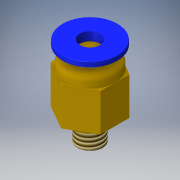
# Autodesk Inventor part: Bowden
Saved by Autodesk Inventor 2016 SP1 (Build 200210100, 210)
## iProperties
Created: 2015-12-27
Part Number: Bowden
Material: Generic
Document SubType Name: Modeling
Designer: Dirk Alferink
Density: 1 g/cm^3
Appearance: Gold
Author: Dirk Alferink
Autodesk Inventor part; units mm, degrees
ref_plane "YZ Plane" through (0, 0, 0) normal (1, 0, 0) x (0, 1, 0)
ref_plane "XZ Plane" through (0, 0, 0) normal (0, 1, 0) x (-1, 0, 0)
ref_plane "XY Plane" through (0, 0, 0) normal (0, 0, 1) x (1, 0, 0)
sketch "Sketch1" plane through (0, 0, 0) normal (0, 1, 0) x (-1, 0, 0)
  line L0 (0, 0) -> (2.5, 0)
  line L1 (2.5, 0) -> (2.5, 4)
  line L2 (2.5, 4) -> (4, 4)
  line L3 (4, 4) -> (4, 5)
  line L4 (4, 5) -> (0, 5)
  line L5 (0, 5) -> (0, 0)
  dimension "d0" = 2.5
  dimension "d1" = 4
  dimension "d2" = 1.5
  constraints: 12 end point, 4 perpendicular, 2 horizontal
  measures "d0" distance of L0.start L0.end
  measures "d1" distance of L0.end L1.end
  measures "d2" distance of L1.end L2.end
revolve "Revolution1" add sketch "Sketch1" angle 360 about axis through (0, 0, 5) along (0, 0, -1)
thread "Thread1" size "M5x0.8" class "6g" standard "ANSI Metric M Profile" full length
sketch "Sketch2" plane through (0, 0, 5) normal (0, 0, 1) x (1, 0, 0)
  line L0 (5, 2.8868) -> (5, -2.8868)
  line L1 (5, -2.8868) -> (0, -5.7735)
  line L2 (0, -5.7735) -> (-5, -2.8868)
  line L3 (-5, -2.8868) -> (-5, 2.8868)
  line L4 (-5, 2.8868) -> (0, 5.7735)
  line L5 (0, 5.7735) -> (5, 2.8868)
  point P0 (0, 0)
  point P1 (0, 0)
  dimension "d9" = 10
  constraints: 12 end point, 1 coincident, 1 vertical alignment, 13 other
  measures "d9" distance between parallel lines of L1 L4
extrude "Extrusion1" add sketch "Sketch2" along normal blind 7.5
sketch "Sketch3" plane through (0, 0, 12.5) normal (0, 0, 1) x (1, 0, 0)
  circle A0 centre (0, 0) radius 5
  dimension "d12" = 10
  constraints: 1 centre point, 1 coincident
  measures "d12" diameter of A0
extrude "Extrusion2" add sketch "Sketch3" along normal blind 2.5
fillet "Fillet1" radius 1.5 1 edges at (-5, 0, 15)
sketch "Sketch4" plane through (0, 0, 15) normal (0, 0, 1) x (1, 0, 0)
  circle A0 centre (0, 0) radius 2.5
  dimension "d16" = 5
  constraints: 1 centre point, 1 coincident
  measures "d16" diameter of A0
extrude "Extrusion3" add sketch "Sketch4" along normal blind 1.5
sketch "Sketch5" plane through (0, 0, 16.5) normal (0, 0, 1) x (1, 0, 0)
  circle A0 centre (0, 0) radius 5.5
  dimension "d19" = 11
  constraints: 1 centre point, 1 coincident
  measures "d19" diameter of A0
extrude "Extrusion4" add sketch "Sketch5" along normal blind 1
sketch "Sketch6" plane through (0, 0, 17.5) normal (0, 0, 1) x (1, 0, 0)
  circle A0 centre (0, 0) radius 2.5 projected
  constraints: 1 coincident
hole "Hole1" at (0, 0, 17.5) direction (0, 0, -1) diameter 4 end through all
fillet "Fillet2" radius 0.1 2 edges at (-5.5, 0, 17.5) (-5.5, 0, 16.5)
fillet "Fillet3" radius 0.2 6 edges at (0, -5.7735, 8.75) (5, -2.8868, 8.75) (5, 2.8868, 8.75) (0, 5.7735, 8.75) (-5, 2.8868, 8.75) (-5, -2.8868, 8.75)
sketch "Sketch7" plane through (0, 0, 15) normal (0, 0, 1) x (1, 0, 0)
  circle A0 centre (0, 0) radius 3.5
  constraints: 1 centre point, 1 coincident
extrude "Extrusion5" add sketch "Sketch7" along normal blind 0.75
body "Solid1"
